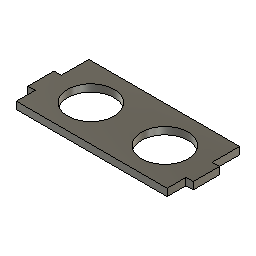
Activity2Solution v1 (Autodesk Fusion 360 design; units mm, degrees)
Autodesk Fusion 360 part; units mm, degrees
sketch "Sketch1" plane through (0, 0, 0) normal (0, 0, 1) x (1, 0, 0)
  line L0 (15, 55) -> (67, 55)
  line L1 (15, 55) -> (15, 45.5)
  line L2 (15, 45.5) -> (12.5, 45.5)
  line L3 (12.5, 45.5) -> (12.5, 36.5)
  line L4 (12.5, 36.5) -> (15, 36.5)
  line L5 (15, 36.5) -> (15, 30)
  line L6 (15, 30) -> (67, 30)
  line L7 (67, 30) -> (67, 36.5)
  line L8 (67, 36.5) -> (69.5, 36.5)
  line L9 (69.5, 36.5) -> (69.5, 45.5)
  line L10 (69.5, 45.5) -> (67, 45.5)
  line L11 (67, 45.5) -> (67, 55)
  circle A0 centre (28.3, 42.4) radius 8
  circle A1 centre (53.8, 42.4) radius 8
  dimension "d1" = 52
  dimension "d2" = 9.5
  dimension "d3" = 2.5
  dimension "d4" = 9
  dimension "d5" = 2.5
  dimension "d6" = 6.5
  dimension "d7" = 52
  dimension "d8" = 6.5
  dimension "d9" = 2.5
  dimension "d10" = 9
  dimension "d11" = 2.5
  dimension "d12" = 16
  dimension "d13" = 16
  dimension "d14" = 12.4
  dimension "d15" = 15.8
  dimension "d16" = 25.5
  dimension "d17" = 12.4
  constraint horizontal L0
  constraint perpendicular L0 L1
  constraint horizontal L2
  constraint perpendicular L2 L3
  constraint perpendicular L3 L4
  constraint perpendicular L4 L5
  constraint perpendicular L5 L6
  constraint perpendicular L6 L7
  constraint perpendicular L7 L8
  constraint perpendicular L8 L9
  constraint perpendicular L9 L10
  measures "d1" distance of L0.start L0.end
  measures "d2" distance of L0.start L1.end
  measures "d3" distance of L1.end L2.end
  measures "d4" distance of L2.end L3.end
  measures "d5" distance of L3.end L4.end
  measures "d6" distance of L4.end L5.end
  measures "d7" distance of L5.end L6.end
  measures "d8" distance of L6.end L7.end
  measures "d9" distance of L7.end L8.end
  measures "d10" distance of L8.end L9.end
  measures "d11" distance of L9.end L10.end
  measures "d12" diameter of A0
  measures "d13" diameter of A1
  measures "d14" distance of L6 A0.centre
  measures "d15" distance of L3 A0.centre
  measures "d16" horizontal distance of A0.centre A1.centre
  measures "d17" distance of L6 A1.centre
extrude "Extrude1" add sketch "Sketch1" along normal blind 2.5
